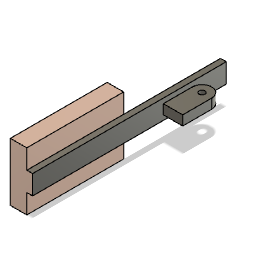
stamp pad v3 (Autodesk Fusion 360 design; units mm, degrees)
Autodesk Fusion 360 part; units mm, degrees
sketch "Sketch1" plane through (0, 0, 0) normal (1, 0, 0) x (0, 0, -1)
  line L0 (-50, 30) -> (50, 30)
  line L1 (50, 30) -> (50, -30)
  line L2 (50, -30) -> (-50, -30)
  line L3 (-50, -30) -> (-50, 30)
  line L4 (48, -28) -> (-48, -28)
  line L5 (-48, -28) -> (-48, 28)
  line L6 (-48, 28) -> (48, 28)
  line L7 (48, 28) -> (48, -28)
  dimension "d1" = 100
  dimension "d2" = 60
  dimension "d3" = 2
  dimension "d17" = 30
  dimension "d18" = 50
  constraint horizontal L0
  constraint perpendicular L0 L1
  constraint parallel L0 L2
  constraint parallel L1 L3
  measures "d1" distance of L1.end L2.end
  measures "d2" distance of L0.end L1.end
  measures "d17" distance of L0 origin
  measures "d18" distance of origin L3
extrude "Extrude1" add sketch "Sketch1" along normal blind 2 contours L0 L1 L2 L3 | L4 L5 L6 L7
extrude "Extrude2" add sketch "Sketch1" against normal blind 15
sketch "Sketch2" plane through (0, 0, 0) normal (-1, 0, 0) x (0, 0, 1)
  line L0 (-48, 28) -> (-48, -28)
  line L1 (-48, -28) -> (48, -28)
  line L2 (48, -28) -> (48, 28)
  line L3 (48, 28) -> (-48, 28)
  line L4 (45, 25) -> (-45, 25)
  line L5 (-45, 25) -> (-45, -25)
  line L6 (-45, -25) -> (45, -25)
  line L7 (45, -25) -> (45, 25)
  line L8 (45, 25) -> (-45, -25) construction
  line L9 (-45, 25) -> (45, -25) construction
  dimension "d8" = 90
  dimension "d9" = 50
  constraint horizontal L4
  constraint perpendicular L4 L5
  constraint parallel L4 L6
  constraint parallel L5 L7
  constraint coincident L8 origin
  constraint coincident L9 origin
  measures "d8" distance of L5.end L6.end
  measures "d9" distance of L4.end L5.end
extrude "Extrude3" add sketch "Sketch2" along normal blind 13 contours L4 L5 L6 L7
sketch "Sketch4" plane through (2, 0, 0) normal (1, 0, 0) x (0, 0, -1)
  line L0 (-50, -30) -> (50, -30)
  line L1 (50, -30) -> (50, 30)
  line L2 (50, 30) -> (-50, 30)
  line L3 (-50, 30) -> (-50, -30)
  line L4 (-50, 10) -> (150, 10)
  line L5 (150, 10) -> (150, -10)
  line L6 (150, -10) -> (-50, -10)
  line L7 (-50, -10) -> (-50, 10)
  constraint horizontal L4
  constraint vertical L5
  constraint horizontal L6
  constraint vertical L7
  constraint coincident L3 L4.start
extrude "Extrude4" add sketch "Sketch4" along normal blind 6 contours L1 L3 L4 L6 L7 | L1 L4 L5 L6
sketch "Sketch5" plane through (0, -10, 0) normal (0, -1, 0) x (1, 0, 0)
  line L0 (2, -50) -> (2, -150)
  line L1 (2, -150) -> (8, -150)
  line L2 (8, -150) -> (8, 50)
  line L3 (8, 50) -> (2, 50)
  line L4 (2, 50) -> (2, -50)
  line L5 (28, -115) -> (28, -85)
  line L6 (28, -85) -> (8, -85)
  arc A0 (8, -115) -> (28, -115) centre (18, -115) ccw
  circle A1 centre (18, -115) radius 3
  dimension "d28" = 6
  constraint vertical L5
  constraint coincident L2 L6.end
  constraint perpendicular L2 L6
  constraint coincident L2 A0.start
  constraint concentric A0 A1
  measures "d28" diameter of A1
extrude "Extrude5" add sketch "Sketch5" against normal blind 10 from surface at -5 contours L2 L5 L6 A0
